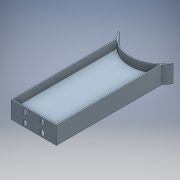
# Autodesk Inventor part: Fix Saddle new 1
Saved by Autodesk Inventor 2016 (Build 200138000, 138)
## iProperties
Created: 2018-11-07
Part Number: Fix Saddle new 1
Material: Steel ASTM A36
Document SubType Name: Modeling
Designer: asus
Density: 7.85 g/cm^3
Appearance: Steel Blue
Mass: 18172.8 g
Surface Area: 6469.58 cm^2
Volume: 2315.01 cm^3
Author: asus
Autodesk Inventor part; units mm, degrees
ref_plane "YZ Plane" through (0, 0, 0) normal (1, 0, 0) x (0, 1, 0)
ref_plane "XZ Plane" through (0, 0, 0) normal (0, 1, 0) x (-1, 0, 0)
ref_plane "XY Plane" through (0, 0, 0) normal (0, 0, 1) x (1, 0, 0)
sketch "Sketch1" plane through (0, 0, 0) normal (0, 0, 1) x (1, 0, 0)
  line L0 (-130, 607) -> (-130, 0)
  line L1 (-130, 0) -> (130, 0)
  line L2 (130, 0) -> (130, 607)
  line L3 (125, 5) -> (125, 602.1317)
  line L4 (-125, 5) -> (-125, 602.1317)
  line L5 (-125, 5) -> (125, 5)
  arc A0 (-153.9793, 646.614) -> (153.9793, 646.614) centre (0, 735.514) ccw
  arc A1 (130, 607) -> (158.3094, 644.114) centre (0, 735.514) ccw
  arc A2 (-158.3094, 644.114) -> (-130, 607) centre (0, 735.514) ccw
  arc A3 (-125, 602.1317) -> (125, 602.1317) centre (0, 735.514) ccw
  line L6 (-158.3094, 644.114) -> (-153.9793, 646.614)
  line L7 (153.9793, 646.614) -> (158.3094, 644.114)
  point P0 (0, 0)
  point P1 (0, 0)
  point P2 (0, 5)
  dimension "d0" = 260
  dimension "d2" = 607
  dimension "d3" = 607
  dimension "d6" = 5
  dimension "d7" = 5
  dimension "d8" = 5
  dimension "d57" = 355.6
  dimension "d61" = 5
  dimension "d64" = 182.8
  dimension "d79" = 130
  dimension "d80" = 120
  dimension "d81" = 158.3094
  dimension "d82" = 153.9793
  dimension "d83" = 153.9793
  constraints: 16 end point, 8 point on circle, 4 centre point, 4 coincident, 3 vertical, 2 midpoint, 2 perpendicular, 1 parallel, 1 vertical alignment
  measures "d0" distance of L0.end L1.end
  measures "d2" distance of L0.start L0.end
  measures "d3" distance of L1.end L2.end
  measures "d6" distance between parallel lines of L0 L4
  measures "d7" distance between parallel lines of L2 L3
  measures "d8" distance between parallel lines of L1 L5
  measures "d57" diameter of A0
  measures "d61" radial gap between concentric circles of A3 A0
  measures "d64" radius of A1
  measures "d79" distance from line of L0 A1.centre
  measures "d80" angle of L7 L6
  measures "d81" horizontal distance of L6.start A0.centre
  measures "d82" horizontal distance of L6.end A0.centre
  measures "d83" horizontal distance of L7.start A0.centre
extrude "Extrusion1" add sketch "Sketch1" along normal mid plane 100
sketch "Sketch5" plane through (0, 0, 0) normal (0, 0, 1) x (1, 0, 0)
  line L0 (-125, 602.1317) -> (-125, 5) projected
  line L1 (-125, 602.1317) -> (-125, 5)
  line L2 (-125, 5) -> (125, 5)
  line L3 (-125, 5) -> (125, 5) projected
  line L4 (125, 5) -> (125, 602.1317) projected
  line L5 (125, 5) -> (125, 602.1317)
  arc A0 (-125, 602.1317) -> (125, 602.1317) centre (0, 735.514) ccw
  point P0 (0, 0)
  point P1 (0, 5)
  dimension "d67" = 365.6
  constraints: 6 end point, 2 collinear, 2 perpendicular, 2 point on circle, 1 centre point, 1 midpoint, 1 vertical alignment
  measures "d67" diameter of A0
extrude "Extrusion2" add sketch "Sketch5" along normal mid plane 10
sketch "Sketch6" plane through (-130, 0, 50) normal (0, -1, 0) x (1, 0, 0)
  line L0 (5, -100) -> (255, -100) projected
  line L1 (130, -100) -> (130, 0)
  line L2 (0, 0) -> (260, 0) projected
  line L3 (80, -16) -> (80, -28.5) construction
  line L4 (70, -16) -> (70, -28.5)
  line L5 (90, -28.5) -> (90, -16)
  arc A0 (90, -16) -> (70, -16) centre (80, -16) ccw
  arc A1 (70, -28.5) -> (90, -28.5) centre (80, -28.5) ccw
  line L6 (80, -71.5) -> (80, -84) construction
  line L7 (70, -71.5) -> (70, -84)
  line L8 (90, -84) -> (90, -71.5)
  arc A2 (90, -71.5) -> (70, -71.5) centre (80, -71.5) ccw
  arc A3 (70, -84) -> (90, -84) centre (80, -84) ccw
  line L9 (180, -16) -> (180, -28.5) construction
  line L10 (190, -16) -> (190, -28.5)
  line L11 (170, -28.5) -> (170, -16)
  arc A4 (190, -16) -> (170, -16) centre (180, -16) ccw
  arc A5 (170, -28.5) -> (190, -28.5) centre (180, -28.5) ccw
  line L12 (180, -71.5) -> (180, -84) construction
  line L13 (190, -71.5) -> (190, -84)
  line L14 (170, -84) -> (170, -71.5)
  arc A6 (190, -71.5) -> (170, -71.5) centre (180, -71.5) ccw
  arc A7 (170, -84) -> (190, -84) centre (180, -84) ccw
  point P0 (130, -50)
  point P1 (80, -22.25)
  point P2 (80, -77.75)
  point P3 (180, -22.25)
  point P4 (180, -77.75)
  dimension "d88" = 100
  dimension "d89" = 10
  dimension "d90" = 100
  dimension "d92" = 10
  dimension "d93" = 68
  dimension "d94" = 16
  dimension "d95" = 43
  dimension "d96" = 12.5
  constraints: 34 end point, 16 point on circle, 14 symmetric about line, 8 centre point, 8 tangent, 4 midpoint, 2 parallel, 2 vertical, 4 other
  measures "d88" diameter of point (80, -22.25) L1
  measures "d89" radius of A0
  measures "d90" diameter of point (80, -77.75) L1
  measures "d92" radius of A2
  measures "d93" distance of L7.end L4.start
  measures "d94" distance from line of L2 L4.start
  measures "d95" distance of L8.end L5.start
  measures "d96" distance of L8.start L8.end
extrude "Extrusion5" cut sketch "Sketch6" against normal blind 10
body "Solid1"
